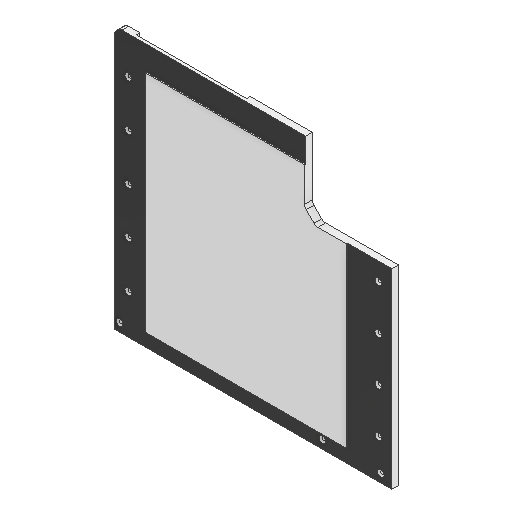
# Autodesk Inventor part: ElectronicsBase
Saved by Autodesk Inventor 2026.2 (Build 302298000, 298)
## iProperties
Created: 2026-01-14
Part Number: ElectronicsBase
Material: ABS Plastic
Document SubType Name: Modeling
Designer: gaoet
Density: 1.06 g/cm^3
Appearance: Smooth - White
Author: gaoet
Autodesk Inventor part; units mm, degrees
ref_plane "YZ Plane" through (0, 0, 0) normal (1, 0, 0) x (0, 1, 0)
ref_plane "XZ Plane" through (0, 0, 0) normal (0, 1, 0) x (-1, 0, 0)
ref_plane "XY Plane" through (0, 0, 0) normal (0, 0, 1) x (1, 0, 0)
sketch "Sketch1" plane through (0, 0, 0) normal (0, 0, 1) x (1, 0, 0)
  line L0 (-125.5, -122) -> (125.5, -122)
  line L1 (125.5, -122) -> (125.5, 122)
  line L2 (125.5, 122) -> (-125.5, 122)
  line L3 (-125.5, 122) -> (-125.5, -122)
  line L4 (-125.5, -122) -> (125.5, 122) construction
  line L5 (125.5, -122) -> (-125.5, 122) construction
  line L6 (125.5, 122) -> (47.5, 122)
  line L7 (47.5, 122) -> (47.5, 51)
  line L8 (47.5, 51) -> (125.5, 51)
  line L9 (125.5, 51) -> (125.5, 122)
  point P0 (0, 0)
  point P1 (125.5, 51)
  dimension "d0" = 251
  dimension "d1" = 244
  dimension "d6" = 78
  dimension "d7" = 71
  constraints: 20 end point, 4 parallel, 2 horizontal, 2 midpoint, 2 perpendicular
  measures "d0" distance of L1.end L2.end
  measures "d1" distance of L2.end L0.start
  measures "d6" distance of L7.end L8.end
  measures "d7" distance of L6.end L7.end
extrude "Extrusion1" add sketch "Sketch1" along normal blind 7 contours L3 L2 L7 L8 L1 L0
sketch "Sketch2" plane through (0, 0, 7) normal (0, 0, 1) x (1, 0, 0)
  line L0 (-100, -100) -> (100, -100)
  line L1 (100, -100) -> (100, 100)
  line L2 (100, 100) -> (-100, 100)
  line L3 (-100, 100) -> (-100, -100)
  line L4 (-100, -100) -> (100, 100) construction
  line L5 (100, -100) -> (-100, 100) construction
  point P0 (0, 0)
  point P1 (0, 0)
  dimension "d4" = 200
  dimension "d5" = 200
  constraints: 12 end point, 2 coincident, 2 midpoint, 2 parallel, 1 horizontal, 1 perpendicular
  measures "d4" distance of L2.end L1.end
  measures "d5" distance of L1.end L0.end
sketch "Sketch3" plane through (0, 0, 7) normal (0, 0, 1) x (1, 0, 0)
  line L0 (-85.5721, 144.9839) -> (-125.5, 112)
  line L1 (-125.5, 122) -> (-125.5, -122) projected
  line L2 (-85.5721, 144.9839) -> (-17.6358, 144.9839) construction
  line L3 (125.5, -122) -> (125.5, 51) projected
  line L4 (125.5, 51) -> (47.5, 51) projected
  line L5 (47.5, 51) -> (47.5, 122) projected
  line L6 (47.5, 122) -> (-125.5, 122) projected
  line L7 (-125.5, 122) -> (-125.5, -122) projected
  line L8 (-125.5, -122) -> (125.5, -122) projected
  point P0 (0, 0)
  point P1 (-113.3947, 122)
  point P2 (-125.5, 122)
  dimension "d9" = 140.44
  dimension "d10" = 10
  constraints: 4 end point, 1 horizontal, 1 point on line
  measures "d9" angle of L0 L2
  measures "d10" distance of L1.start L0.end
extrude "Extrusion2" cut sketch "Sketch3" against normal blind 10 contours L0 L1 L6
fillet "Fillet1" radius 5 2 edges at (-113.3947, 122, 3.5) (-125.5, 112, 3.5)
chamfer "Chamfer1" distance 10 angle 45 1 edges at (47.5, 51, 3.5)
sketch "Sketch4" plane through (0, 0, 7) normal (0, 0, 1) x (1, 0, 0)
  line L0 (-125.5, 109.645) -> (-125.5, -122) projected
  line L1 (125.5, -122) -> (125.5, 51) projected
  line L2 (-125.5, -122) -> (125.5, -122) projected
  point P0 (0, 0)
  point P1 (-121, -114.5)
  point P2 (115.5, -114.5)
  point P3 (10, -114.5)
  point P4 (62.75, -114.5)
  dimension "d17" = 4.5
  dimension "d20" = 10
  dimension "d21" = 7.5
  dimension "d42" = 52.75
  dimension "d43" = 52.75
  constraints: 3 horizontal alignment
  measures "d17" distance from line of L0 point (-121, -114.5)
  measures "d20" distance from line of L1 point (115.5, -114.5)
  measures "d21" distance from line of L2 point (-121, -114.5)
  measures "d42" distance of point (62.75, -114.5) point (10, -114.5)
  measures "d43" distance of point (115.5, -114.5) point (62.75, -114.5)
hole "Hole1" at (-121, -114.5, 7) at (115.5, -114.5, 7) at (62.75, -114.5, 7) direction (0, 0, -1) diameter 3 depth 15 countersink diameter 6 countersink angle 100
sketch "Sketch5" plane through (0, 0, 7) normal (0, 0, 1) x (1, 0, 0)
  line L0 (-96.82, 94.1) -> (85.02, 94.1)
  line L1 (85.02, 94.1) -> (85.02, -109.4)
  line L2 (85.02, -109.4) -> (-96.82, -109.4)
  line L3 (-96.82, -109.4) -> (-96.82, 94.1)
  line L4 (125.5, -122) -> (125.5, 51) projected
  line L5 (-125.5, 109.645) -> (-125.5, -122) projected
  line L6 (47.5, 122) -> (-111.5966, 122) projected
  line L7 (-125.5, -122) -> (125.5, -122) projected
  circle A0 centre (115.5, -114.5) radius 3 projected
  circle A1 centre (-121, -114.5) radius 3 projected
  arc A2 (-123.6844, 113.4998) -> (-125.5, 109.645) centre (-120.5, 109.645) ccw projected
  line L8 (-125.5, 109.645) -> (-125.5, -122) projected
  line L9 (-125.5, -122) -> (125.5, -122) projected
  line L10 (125.5, -122) -> (125.5, 51) projected
  line L11 (125.5, 51) -> (57.5, 51) projected
  line L12 (47.5, 61) -> (57.5, 51) projected
  line L13 (47.5, 61) -> (47.5, 122) projected
  line L14 (47.5, 122) -> (-111.5966, 122) projected
  arc A3 (-111.5966, 122) -> (-114.781, 120.8548) centre (-111.5966, 117) ccw projected
  line L15 (-114.781, 120.8548) -> (-123.6844, 113.4998) projected
  point P0 (0, 0)
  point P1 (47.5, 94.1)
  point P2 (-111.5966, 122)
  point P3 (85.02, 51)
  dimension "d29" = 40.48
  dimension "d30" = 28.68
  dimension "d31" = 27.9
  dimension "d32" = 12.6
  constraints: 8 end point, 2 parallel, 1 horizontal, 1 perpendicular
  measures "d29" distance between parallel lines of L4 L1
  measures "d30" distance between parallel lines of L5 L3
  measures "d31" distance between parallel lines of L6 L0
  measures "d32" distance between parallel lines of L7 L2
extrude "Extrusion3" cut sketch "Sketch5" against normal blind 1 contours L3 L2 L1 L11 L4 L7 L5 A2 L15 A3 L6 L13 L0 | A0 | A1
sketch "Sketch6" plane through (0, 0, 6) normal (0, 0, 1) x (1, 0, 0)
  circle A0 centre (115.5, -114.5) radius 1.8082 projected
  circle A1 centre (-121, -114.5) radius 1.8082 projected
  line L0 (47.5, 94.1) -> (-96.82, 94.1) projected
  line L1 (47.5, 122) -> (47.5, 94.1) projected
  line L2 (-111.5966, 122) -> (47.5, 122) projected
  arc A2 (-111.5966, 122) -> (-114.781, 120.8548) centre (-111.5966, 117) ccw projected
  line L3 (-123.6844, 113.4998) -> (-114.781, 120.8548) projected
  arc A3 (-123.6844, 113.4998) -> (-125.5, 109.645) centre (-120.5, 109.645) ccw projected
  line L4 (-125.5, -122) -> (-125.5, 109.645) projected
  line L5 (125.5, -122) -> (-125.5, -122) projected
  line L6 (125.5, 51) -> (125.5, -122) projected
  line L7 (85.02, 51) -> (125.5, 51) projected
  line L8 (85.02, -109.4) -> (85.02, 51) projected
  line L9 (-96.82, -109.4) -> (85.02, -109.4) projected
  line L10 (-96.82, 94.1) -> (-96.82, -109.4) projected
  circle A4 centre (62.75, -114.5) radius 1.8082 projected
  circle A5 centre (115.5, -114.5) radius 1.8082 projected
  circle A6 centre (-121, -114.5) radius 1.8082 projected
  line L11 (47.5, 94.1) -> (-96.82, 94.1) projected
  line L12 (47.5, 122) -> (47.5, 94.1) projected
  line L13 (-111.5966, 122) -> (47.5, 122) projected
  arc A7 (-111.5966, 122) -> (-114.781, 120.8548) centre (-111.5966, 117) ccw projected
  line L14 (-123.6844, 113.4998) -> (-114.781, 120.8548) projected
  arc A8 (-123.6844, 113.4998) -> (-125.5, 109.645) centre (-120.5, 109.645) ccw projected
  line L15 (-125.5, -122) -> (-125.5, 109.645) projected
  line L16 (125.5, -122) -> (-125.5, -122) projected
  line L17 (125.5, 51) -> (125.5, -122) projected
  line L18 (85.02, 51) -> (125.5, 51) projected
  line L19 (85.02, -109.4) -> (85.02, 51) projected
  line L20 (-96.82, -109.4) -> (85.02, -109.4) projected
  line L21 (-96.82, 94.1) -> (-96.82, -109.4) projected
  point P0 (0, 0)
hole "Hole2" at (-121, -114.5, 6) at (115.5, -114.5, 6) at (62.75, -114.5, 6) direction (0, 0, -1) diameter 3 depth 15 countersink diameter 6 countersink angle 100
sketch "Sketch7" plane through (0, 0, 6) normal (0, 0, 1) x (1, 0, 0)
  circle A0 centre (62.75, -114.5) radius 3 projected
  circle A1 centre (115.5, -114.5) radius 3 projected
  circle A2 centre (-121, -114.5) radius 3 projected
  line L0 (47.5, 94.1) -> (-96.82, 94.1) projected
  line L1 (47.5, 122) -> (47.5, 94.1) projected
  line L2 (-111.5966, 122) -> (47.5, 122) projected
  arc A3 (-111.5966, 122) -> (-114.781, 120.8548) centre (-111.5966, 117) ccw projected
  line L3 (-123.6844, 113.4998) -> (-114.781, 120.8548) projected
  arc A4 (-123.6844, 113.4998) -> (-125.5, 109.645) centre (-120.5, 109.645) ccw projected
  line L4 (-125.5, -122) -> (-125.5, 109.645) projected
  line L5 (125.5, -122) -> (-125.5, -122) projected
  line L6 (125.5, 51) -> (125.5, -122) projected
  line L7 (85.02, 51) -> (125.5, 51) projected
  line L8 (85.02, -109.4) -> (85.02, 51) projected
  line L9 (-96.82, -109.4) -> (85.02, -109.4) projected
  line L10 (-96.82, 94.1) -> (-96.82, -109.4) projected
  point P0 (0, 0)
  point P1 (113.25, 34.75)
  point P2 (113.25, -5.75)
  point P3 (113.25, -46.25)
  point P4 (113.25, -86.75)
  point P5 (-113.25, -86)
  point P6 (-113.25, -44)
  point P7 (-113.25, -2)
  point P8 (-113.25, 40)
  point P9 (-113.25, 82)
  dimension "d44" = 12.25
  dimension "d45" = 35.25
  dimension "d46" = 40.5
  dimension "d47" = 40.5
  dimension "d48" = 40.5
  dimension "d56" = 36
  dimension "d57" = 42
  dimension "d58" = 42
  dimension "d59" = 42
  dimension "d60" = 42
  dimension "d61" = 12.25
  constraints: 7 vertical alignment
  measures "d44" distance from line of L6 point (113.25, -86.75)
  measures "d45" distance from line of L5 point (113.25, -86.75)
  measures "d46" distance of point (113.25, -86.75) point (113.25, -46.25)
  measures "d47" distance of point (113.25, -46.25) point (113.25, -5.75)
  measures "d48" distance of point (113.25, -5.75) point (113.25, 34.75)
  measures "d56" distance from line of L5 point (-113.25, -86)
  measures "d57" distance of point (-113.25, -86) point (-113.25, -44)
  measures "d58" distance of point (-113.25, -44) point (-113.25, -2)
  measures "d59" distance of point (-113.25, -2) point (-113.25, 40)
  measures "d60" distance of point (-113.25, 40) point (-113.25, 82)
  measures "d61" distance from line of L4 point (-113.25, -86)
hole "Hole3" at (113.25, 34.75, 6) at (113.25, -5.75, 6) at (113.25, -46.25, 6) at (113.25, -86.75, 6) at (-113.25, 82, 6) at (-113.25, 40, 6) at (-113.25, -2, 6) at (-113.25, -44, 6) at (-113.25, -86, 6) direction (0, 0, -1) diameter 3 depth 10 countersink diameter 6 countersink angle 100
sketch "Sketch8" plane through (0, 0, 0) normal (0, 0, -1) x (-1, 0, 0)
  circle A0 centre (113.25, -86) radius 1.5 projected
  circle A1 centre (113.25, -44) radius 1.5 projected
  circle A2 centre (113.25, -2) radius 1.5 projected
  circle A3 centre (113.25, 40) radius 1.5 projected
  circle A4 centre (113.25, 82) radius 1.5 projected
  circle A5 centre (-113.25, -86.75) radius 1.5 projected
  circle A6 centre (-113.25, -46.25) radius 1.5 projected
  circle A7 centre (-113.25, -5.75) radius 1.5 projected
  circle A8 centre (-113.25, 34.75) radius 1.5 projected
  circle A9 centre (-62.75, -114.5) radius 1.5 projected
  circle A10 centre (-115.5, -114.5) radius 1.5 projected
  circle A11 centre (121, -114.5) radius 1.5 projected
  arc A12 (125.5, 109.645) -> (123.6844, 113.4998) centre (120.5, 109.645) ccw projected
  line L0 (123.6844, 113.4998) -> (114.781, 120.8548) projected
  arc A13 (114.781, 120.8548) -> (111.5966, 122) centre (111.5966, 117) ccw projected
  line L1 (-47.5, 122) -> (111.5966, 122) projected
  line L2 (-47.5, 61) -> (-47.5, 122) projected
  line L3 (-57.5, 51) -> (-47.5, 61) projected
  line L4 (-125.5, 51) -> (-57.5, 51) projected
  line L5 (-125.5, -122) -> (-125.5, 51) projected
  line L6 (125.5, -122) -> (-125.5, -122) projected
  line L7 (125.5, 109.645) -> (125.5, -122) projected
  line L8 (108.75, 122) -> (108.75, -122)
  line L9 (8.75, 122) -> (8.75, -122)
  line L10 (108.75, -112) -> (8.75, -112)
  point P0 (0, 0)
  dimension "d62" = 4.5
  dimension "d63" = 100
  dimension "d66" = 10
  constraints: 6 end point, 6 point on line, 2 vertical, 1 parallel
  measures "d62" distance from line of L8 A1.centre
  measures "d63" distance between parallel lines of L8 L9
  measures "d66" distance between parallel lines of L10 L6
extrude "Extrusion4" cut sketch "Sketch8" against normal blind 3.25 contours L10 L9 L1 L8
fillet "Fillet2" radius 5 2 edges at (47.5, 61, 3.5) (57.5, 51, 3.5)
sketch "Sketch9" plane through (0, 0, 6) normal (0, 0, 1) x (1, 0, 0)
  circle A0 centre (-113.25, -86) radius 3 projected
  circle A1 centre (-113.25, -44) radius 3 projected
  circle A2 centre (-113.25, -2) radius 3 projected
  circle A3 centre (-113.25, 40) radius 3 projected
  circle A4 centre (-113.25, 82) radius 3 projected
  circle A5 centre (113.25, -86.75) radius 3 projected
  circle A6 centre (113.25, -46.25) radius 3 projected
  circle A7 centre (113.25, -5.75) radius 3 projected
  circle A8 centre (113.25, 34.75) radius 3 projected
  circle A9 centre (62.75, -114.5) radius 3 projected
  circle A10 centre (115.5, -114.5) radius 3 projected
  circle A11 centre (-121, -114.5) radius 3 projected
  line L0 (47.5, 94.1) -> (-96.82, 94.1) projected
  line L1 (47.5, 122) -> (47.5, 94.1) projected
  line L2 (-111.5966, 122) -> (47.5, 122) projected
  arc A12 (-111.5966, 122) -> (-114.781, 120.8548) centre (-111.5966, 117) ccw projected
  line L3 (-123.6844, 113.4998) -> (-114.781, 120.8548) projected
  arc A13 (-123.6844, 113.4998) -> (-125.5, 109.645) centre (-120.5, 109.645) ccw projected
  line L4 (-125.5, -122) -> (-125.5, 109.645) projected
  line L5 (125.5, -122) -> (-125.5, -122) projected
  line L6 (125.5, 51) -> (125.5, -122) projected
  line L7 (85.02, 51) -> (125.5, 51) projected
  line L8 (85.02, -109.4) -> (85.02, 51) projected
  line L9 (-96.82, -109.4) -> (85.02, -109.4) projected
  line L10 (-96.82, 94.1) -> (-96.82, -109.4) projected
  line L11 (47.5, 116) -> (-120.6579, 116)
  point P0 (0, 0)
  dimension "d68" = 6
  constraints: 2 end point, 2 point on line, 1 horizontal
  measures "d68" distance between parallel lines of L2 L11
extrude "Extrusion5" cut sketch "Sketch9" against normal through all contours L11 L3 A12 L2 L1
fillet "Fillet3" radius 5 1 edges at (-120.6579, 116, 3)
equation "\"d43\" = d42"
equation "\"d47\" = d46"
equation "\"d48\" = d47"
equation "\"d58\" = d57"
equation "\"d59\" = d58"
equation "\"d60\" = d59"
equation "\"d61\" = d44"
body "Solid1"
